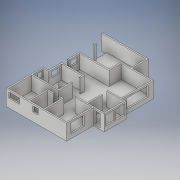
# Autodesk Inventor part: Erdgeschoss
Saved by Autodesk Inventor 2019 (Build 230136000, 136)
## iProperties
Created: 2019-04-30
Part Number: Erdgeschoss
Material: Generisch
Document SubType Name: Modeling
Designer: niede
Density: 1 g/cm^3
Appearance: Vorgabe
Author: niede
Autodesk Inventor part; units mm, degrees
ref_plane "YZ Plane" through (0, 0, 0) normal (1, 0, 0) x (0, 1, 0)
ref_plane "XZ Plane" through (0, 0, 0) normal (0, 1, 0) x (-1, 0, 0)
ref_plane "XY Plane" through (0, 0, 0) normal (0, 0, 1) x (1, 0, 0)
sketch "Skizze1" plane through (0, 0, 0) normal (0, 1, 0) x (-1, 0, 0)
  line L0 (0, 0) -> (11230, 0)
  line L1 (11230, 0) -> (11230, -6920)
  line L2 (11230, -6920) -> (10230, -6920)
  line L3 (10230, -6920) -> (10230, -17740)
  line L4 (10230, -17740) -> (11230, -17740)
  line L5 (11230, -17740) -> (11230, -17980)
  line L6 (11230, -17980) -> (2740, -17980)
  line L7 (2740, -17980) -> (2740, -14980)
  line L8 (2740, -14980) -> (-1250, -14980)
  line L9 (-1250, -14980) -> (-1250, -9110)
  line L10 (-1250, -9110) -> (-2000, -9110)
  line L11 (-2000, -9110) -> (-2000, -5010)
  line L12 (-2000, -5010) -> (0, -5010)
  line L13 (0, -5010) -> (0, 0)
  dimension "d0" = 11230
  dimension "d1" = 6920
  dimension "d2" = 1000
  dimension "d3" = 10820
  dimension "d4" = 1000
  dimension "d5" = 240
  dimension "d6" = 8490
  dimension "d11" = 3000
  dimension "d12" = 3990
  dimension "d13" = 5870
  dimension "d14" = 750
  dimension "d15" = 4100
  dimension "d16" = 2000
  constraints: 28 end point, 8 perpendicular, 2 point on line, 2 vertical, 1 horizontal
  measures "d0" distance of L0.start L0.end
  measures "d1" distance of L0.end L1.end
  measures "d2" distance of L1.end L2.end
  measures "d3" distance of L2.end L3.end
  measures "d4" distance of L3.end L4.end
  measures "d5" distance of L4.end L5.end
  measures "d6" distance of L5.end L6.end
  measures "d11" distance of L6.end L7.end
  measures "d12" distance of L7.end L8.end
  measures "d13" distance of L8.end L9.end
  measures "d14" distance of L9.end L10.end
  measures "d15" distance of L10.end L11.end
  measures "d16" distance of L11.end L12.end
extrude "Fundament" add sketch "Skizze1" along normal blind 300
sketch "Skizze3" plane through (0, 300, 0) normal (0, 1, 0) x (1, 0, 0)
  line L0 (0, 5010) -> (2000, 5010) projected
  line L1 (2000, 5010) -> (2000, 9110) projected
  line L2 (2000, 9110) -> (1250, 9110) projected
  line L3 (1250, 9110) -> (1250, 14980) projected
  line L4 (1250, 14980) -> (-2740, 14980) projected
  line L5 (-11230, 0) -> (0, 0)
  line L6 (0, 0) -> (0, 5010)
  line L7 (-240, 5010) -> (-1180.225, 5010)
  line L8 (-1180.225, 5250) -> (-1180.225, 7900)
  line L9 (-1180.225, 8900) -> (1250, 8900)
  line L10 (1250, 9110) -> (1250, 14980)
  line L11 (-2740, 14980) -> (-2740, 17980)
  line L12 (-2740, 17980) -> (-11230, 17980)
  line L13 (-10230, 6920) -> (-11230, 6920)
  line L14 (-11230, 6920) -> (-11230, 0)
  line L15 (-11230, 0) -> (-11230, 6920)
  line L16 (-11230, 0) -> (-11230, 6920)
  line L17 (-11230, 6920) -> (-10230, 6920)
  line L18 (-10230, 17740) -> (-11230, 17740)
  line L19 (-10230, 17740) -> (-11230, 17740)
  line L20 (-11230, 17980) -> (-2740, 17980)
  line L21 (-11230, 17740) -> (-11230, 17980)
  line L22 (-11230, 17980) -> (-2740, 17980)
  line L23 (-2740, 17980) -> (-2740, 14980)
  line L24 (1250, 14980) -> (1250, 9110)
  line L25 (-1180.225, 7900) -> (-1180.225, 5250)
  line L26 (0, 5010) -> (0, 0)
  line L27 (0, 0) -> (-11230, 0)
  line L28 (-240, 240) -> (-240, 5010)
  line L29 (-1420.225, 5250) -> (-1420.225, 7900)
  line L30 (-1420.225, 7900) -> (-1180.225, 7900)
  line L31 (-9990, 17740) -> (-6230, 17740)
  line L32 (-5990, 17740) -> (-2980, 17740)
  line L33 (-2980, 17740) -> (-2980, 14980)
  line L34 (-2980, 14740) -> (1010, 14740)
  line L35 (1010, 14740) -> (1010, 9140)
  line L36 (1010, 9140) -> (-1420.225, 9140)
  line L37 (-1420.225, 9140) -> (-1420.225, 8900)
  line L38 (-1420.225, 8900) -> (-952.7911, 8900)
  line L39 (-3420.225, 4770) -> (-3420.225, 5010)
  line L40 (-3420.225, 5010) -> (-2980, 5010)
  line L41 (-10990, 4530) -> (-6230, 4530)
  line L42 (-6230, 4530) -> (-5990, 4530)
  line L43 (-10990, 4770) -> (-6230, 4770)
  line L44 (-6990, 240) -> (-6990, 3530)
  line L45 (-6990, 3530) -> (-5990, 3530)
  line L46 (-5990, 3530) -> (-5990, 3770)
  line L47 (-5990, 3770) -> (-7230, 3770)
  line L48 (-7230, 3770) -> (-7230, 240)
  line L49 (-4480, 240) -> (-4480, 3530)
  line L50 (-4480, 3530) -> (-4990, 3530)
  line L51 (-4990, 3530) -> (-4990, 3770)
  line L52 (-4990, 3770) -> (-4240, 3770)
  line L53 (-4240, 3770) -> (-4240, 240)
  line L54 (-10990, 6680) -> (-9990, 6680)
  line L55 (-10230, 6920) -> (-10230, 17740) projected
  line L56 (-10230, 6920) -> (-10230, 9350)
  line L57 (-10230, 9350) -> (-5990, 9350)
  line L58 (-5990, 9350) -> (-5990, 8600)
  line L59 (-5990, 8600) -> (-6230, 8600)
  line L60 (-6230, 8600) -> (-6230, 9110)
  line L61 (-6230, 9110) -> (-9990, 9110)
  line L62 (-9990, 9110) -> (-9990, 6680)
  line L63 (-5990, 4530) -> (-5990, 7100)
  line L64 (-5990, 7100) -> (-5991.4024, 7100)
  line L65 (-5991.4024, 7100) -> (-5991.4024, 4770)
  line L66 (-8610, 4770) -> (-8610, 6270)
  line L67 (-8610, 6270) -> (-8370, 6270)
  line L68 (-8370, 6270) -> (-8370, 4770)
  line L69 (-6230, 6175) -> (-7370, 6175)
  line L70 (-7370, 6175) -> (-7370, 5935)
  line L71 (-7370, 5935) -> (-6230, 5935)
  line L72 (2000, 9110) -> (2000, 5010) projected
  line L73 (0, 5010) -> (2000, 5010)
  line L74 (2000, 5010) -> (2000, 9110)
  line L75 (1250, 9110) -> (2000, 9110) projected
  line L76 (2000, 9110) -> (1250, 9110)
  line L77 (-1180.225, 5010) -> (-1420.225, 5010)
  line L78 (-3420.225, 5010) -> (-3420.225, 5250)
  line L79 (-3420.225, 5250) -> (-1420.225, 5250)
  line L80 (-1420.225, 5010) -> (-3420.225, 5010)
  line L81 (1250, 8900) -> (1760, 8900)
  line L82 (1760, 8900) -> (1760, 5250)
  line L83 (1760, 5250) -> (-1180.225, 5250)
  line L84 (-2740, 14980) -> (1250, 14980)
  line L85 (-10230, 17740) -> (-10230, 6920) projected
  line L86 (-9990, 12449.8635) -> (-4540, 12449.8635)
  line L87 (-4540, 12449.8635) -> (-4540, 14740)
  line L88 (-4540, 14740) -> (-2980, 14740)
  line L89 (-10230, 12689.8635) -> (-4780, 12689.8635)
  line L90 (-4780, 12689.8635) -> (-4780, 14980)
  line L91 (-4780, 14980) -> (-2980, 14980)
  line L92 (-10230, 15189.8635) -> (-9990, 15189.8635)
  line L93 (-9990, 15189.8635) -> (-9990, 15589.8635)
  line L94 (-9990, 15589.8635) -> (-10230, 15589.8635)
  line L95 (-10230, 15589.8635) -> (-10230, 15189.8635)
  line L96 (-10230, 12449.8635) -> (-10230, 10350)
  line L97 (-9990, 10350) -> (-9990, 12449.8635)
  line L98 (-9990, 10350) -> (-10230, 10350)
  line L99 (-10990, 240) -> (-7230, 240)
  line L100 (-6990, 240) -> (-4480, 240)
  line L101 (-4240, 240) -> (-240, 240)
  line L102 (-10990, 240) -> (-10990, 4530)
  line L103 (-10990, 4770) -> (-10990, 6680)
  line L104 (-6230, 4770) -> (-6230, 5935)
  line L105 (-6230, 6175) -> (-6230, 7100)
  line L106 (-6230, 7100) -> (-5991.4024, 7100)
  line L107 (-10230, 12449.8635) -> (-10230, 12689.8635)
  line L108 (-9990, 17740) -> (-10230, 17740)
  line L109 (-5990, 17740) -> (-6230, 17740)
  dimension "d22" = 240
  dimension "d24" = 240
  dimension "d25" = 1000
  dimension "d26" = 240
  dimension "d27" = 240
  dimension "d28" = 240
  dimension "d30" = 240
  dimension "d31" = 240
  dimension "d33" = 240
  dimension "d42" = 240
  dimension "d43" = 240
  dimension "d44" = 240
  dimension "d45" = 240
  dimension "d47" = 2510
  dimension "d48" = 1000
  dimension "d49" = 1000
  dimension "d50" = 240
  dimension "d51" = 240
  dimension "d52" = 90
  dimension "d55" = 2202.7911
  dimension "d56" = 7480
  dimension "d57" = 2430
  dimension "d58" = 750
  dimension "d59" = 240
  dimension "d60" = 240
  dimension "d61" = 240
  dimension "d62" = 1500
  dimension "d63" = 1500
  dimension "d64" = 240
  dimension "d65" = 1000
  dimension "d66" = 240
  dimension "d67" = 240
  dimension "d68" = 240
  dimension "d69" = 240
  dimension "d70" = 240
  dimension "d71" = 5870
  dimension "d72" = 240
  dimension "d73" = 240
  dimension "d74" = 5690
  dimension "d75" = 240
  dimension "d76" = 5050.1365
  dimension "d77" = 2500
  dimension "d78" = 400
  dimension "d79" = 240
  dimension "d80" = 1000
  dimension "d81" = 90
  dimension "d82" = 90
  dimension "d83" = 90
  dimension "d84" = 30
  dimension "d85" = 3860
  dimension "d86" = 8870
  dimension "d87" = 9110
  dimension "d88" = 2010
  dimension "d89" = 5580
  dimension "d90" = 2935
  dimension "d91" = 2190
  dimension "d92" = 750
  dimension "d93" = 2000
  dimension "d94" = 3180.225
  dimension "d95" = 3420.225
  dimension "d96" = 4740
  dimension "d97" = 5420.225
  dimension "d98" = 6240
  dimension "d99" = 6540
  constraints: 202 end point, 50 perpendicular, 16 point on line, 9 horizontal, 8 collinear, 8 vertical, 6 parallel, 1 midpoint, 5 other
  measures "d22" distance between parallel lines of L6 L28
  measures "d24" distance between parallel lines of L8 L29
  measures "d25" distance between parallel lines of L30 L38
  measures "d26" distance between parallel lines of L9 L36
  measures "d27" distance of L9.start L37.end
  measures "d28" distance between parallel lines of L10 L35
  measures "d30" distance between parallel lines of L11 L33
  measures "d31" distance between parallel lines of L12 L32
  measures "d33" distance between parallel lines of L12 L31
  measures "d42" distance of L39.start L39.end
  measures "d43" distance between parallel lines of L53 L49
  measures "d44" distance between parallel lines of L44 L48
  measures "d45" distance between parallel lines of L47 L45
  measures "d47" distance between parallel lines of L44 L49
  measures "d48" distance of L50.end L45.end
  measures "d49" distance of L44.end L45.end
  measures "d50" distance between parallel lines of L43 L41
  measures "d51" distance between parallel lines of L13 L54
  measures "d52" angle of L40 L10
  measures "d55" distance from line of L38.end L10
  measures "d56" distance from line of L41.end L10
  measures "d57" distance of L55.start L56.end
  measures "d58" distance of L57.end L58.end
  measures "d59" distance between parallel lines of L57 L61
  measures "d60" distance between parallel lines of L56 L62
  measures "d61" distance between parallel lines of L60 L58
  measures "d62" distance of L58.end L63.end
  measures "d63" distance of L66.start L66.end
  measures "d64" distance of L66.end L67.end
  measures "d65" distance between parallel lines of L68 L70
  measures "d66" distance between parallel lines of L69 L71
  measures "d67" distance of L39.end L78.end
  measures "d68" distance between parallel lines of L0 L83
  measures "d69" distance between parallel lines of L1 L82
  measures "d70" distance between parallel lines of L4 L34
  measures "d71" distance of L24.start L10.start
  measures "d72" distance between parallel lines of L91 L88
  measures "d73" distance between parallel lines of L87 L90
  measures "d74" distance of L96.start L86.end
  measures "d75" distance between parallel lines of L86 L89
  measures "d76" distance between parallel lines of L31 L89
  measures "d77" distance between parallel lines of L89 L92
  measures "d78" distance of L92.end L93.end
  measures "d79" distance of L92.start L92.end
  measures "d80" distance between parallel lines of L57 L98
  measures "d81" angle of L1 L7
  measures "d82" angle of L75 L39
  measures "d83" angle of L75 L21
  measures "d84" distance between parallel lines of L2 L36
  measures "d85" distance between parallel lines of L2 L79
  measures "d86" distance between parallel lines of L2 L12
  measures "d87" distance between parallel lines of L2 L27
  measures "d88" distance between parallel lines of L2 L64
  measures "d89" distance between parallel lines of L2 L45
  measures "d90" distance between parallel lines of L2 L69
  measures "d91" distance between parallel lines of L2 L13
  measures "d92" distance between parallel lines of L72 L10
  measures "d93" distance between parallel lines of L72 L26
  measures "d94" distance between parallel lines of L72 L8
  measures "d95" distance between parallel lines of L72 L37
  measures "d96" distance between parallel lines of L72 L23
  measures "d97" distance between parallel lines of L72 L78
  measures "d98" distance between parallel lines of L72 L53
  measures "d99" distance between parallel lines of L72 L87
extrude "Wände" add sketch "Skizze3" along normal blind 2600 contours L6 L5 L14 L13 L55 L57 L58 L59 L60 L61 L62 L54 L103 L43 L104 L71 L70 L69 L105 L106 L64 L63 L42 L41 L102 L99 L48 L47 L46 L45 L44 L100 L49 L50 L51 L52 L53 L101 L28 L7 L77 L80 L40 L78 L79 L29 L30 L8 L83 L82 L81 L9 L38 L37 L36 L35 L34 L88 L87 L86 L97 L98 L89 L90 L91 L33 L32 L109 L31 L108 L18 L21 L12 L11 L4 L3 L2 L1 L0 | L55 L94 L93 L92
sketch "Skizze4" plane through (-11230, 0, 0) normal (0, 0, 1) x (1, 0, 0)
  line L0 (500, 2600) -> (2500, 2600)
  line L1 (2500, 2600) -> (2500, 1600)
  line L2 (2500, 1600) -> (500, 1600)
  line L3 (500, 1600) -> (500, 2600)
  line L4 (5000, 2600) -> (6000, 2600)
  line L5 (6000, 2600) -> (6000, 1600)
  line L6 (6000, 1600) -> (5000, 1600)
  line L7 (5000, 1600) -> (5000, 2600)
  line L8 (0, 2900) -> (11230, 2900) projected
  line L9 (0, 0) -> (0, 2900) projected
  dimension "d191" = 2500
  dimension "d192" = 1000
  dimension "d193" = 300
  dimension "d194" = 1000
  dimension "d195" = 2000
  dimension "d196" = 500
  constraints: 16 end point, 4 parallel, 2 horizontal, 2 perpendicular, 2 point on line
  measures "d191" distance between parallel lines of L7 L1
  measures "d192" distance of L2.end L0.start
  measures "d193" distance between parallel lines of L8 L4
  measures "d194" distance of L5.end L6.end
  measures "d195" distance of L1.end L2.end
  measures "d196" distance between parallel lines of L9 L3
extrude "Fenster_West" cut sketch "Skizze4" against normal blind 240
sketch "Skizze5" plane through (0, 0, 0) normal (1, 0, 0) x (0, 0, -1)
  line L0 (0, 2900) -> (5010, 2900) projected
  line L1 (0, 0) -> (0, 2900) projected
  line L2 (800, 2600) -> (3300, 2600)
  line L3 (3300, 2600) -> (3300, 800)
  line L4 (3300, 800) -> (800, 800)
  line L5 (800, 800) -> (800, 2600)
  dimension "d140" = 800
  dimension "d141" = 300
  dimension "d142" = 1800
  dimension "d143" = 2500
  constraints: 8 end point, 2 parallel, 1 horizontal, 1 perpendicular
  measures "d140" distance between parallel lines of L1 L5
  measures "d141" distance between parallel lines of L0 L2
  measures "d142" distance of L4.end L2.start
  measures "d143" distance of L3.end L4.end
extrude "Fenster_Süd_1" cut sketch "Skizze5" against normal blind 240
sketch "Skizze6" plane through (1250, 0, -9110) normal (1, 0, 0) x (0, 0, -1)
  line L0 (830, 2600) -> (4830, 2600)
  line L1 (4830, 2600) -> (4830, 800)
  line L2 (4830, 800) -> (830, 800)
  line L3 (830, 800) -> (830, 2600)
  line L4 (30, 300) -> (30, 2900) projected
  line L5 (0, 2900) -> (5870, 2900) projected
  point P0 (-9110, 0)
  dimension "d146" = 800
  dimension "d147" = 1800
  dimension "d148" = 4000
  dimension "d197" = 300
  constraints: 8 end point, 2 parallel, 1 horizontal, 1 perpendicular
  measures "d146" distance between parallel lines of L4 L3
  measures "d147" distance of L2.end L0.start
  measures "d148" distance of L1.end L2.end
  measures "d197" distance between parallel lines of L5 L0
extrude "Fenster_Süd_2" cut sketch "Skizze6" against normal blind 240
sketch "Skizze7" plane through (0, 0, -5010) normal (0, 0, 1) x (1, 0, 0)
  line L0 (0, 2900) -> (2000, 2900) projected
  line L1 (0, 0) -> (0, 2900) projected
  line L2 (250, 2600) -> (1250, 2600)
  line L3 (1250, 2600) -> (1250, 300)
  line L4 (1250, 300) -> (250, 300)
  line L5 (250, 300) -> (250, 2600)
  line L6 (-1180.225, 300) -> (1760, 300) projected
  dimension "d162" = 250
  dimension "d163" = 1000
  dimension "d165" = 300
  constraints: 8 end point, 2 parallel, 1 collinear, 1 horizontal, 1 perpendicular
  measures "d162" distance between parallel lines of L1 L5
  measures "d163" distance of L2.start L2.end
  measures "d165" distance between parallel lines of L0 L2
extrude "Fenster_Wintergarten_1" cut sketch "Skizze7" against normal blind 240
sketch "Skizze8" plane through (2000, 0, -5010) normal (1, 0, 0) x (0, 0, -1)
  line L0 (4100, 0) -> (4100, 2900) projected
  line L1 (0, 2900) -> (4100, 2900) projected
  line L2 (0, 0) -> (0, 2900) projected
  line L3 (240, 2600) -> (1930, 2600)
  line L4 (1930, 2600) -> (1930, 800)
  line L5 (1930, 800) -> (240, 800)
  line L6 (240, 800) -> (240, 2600)
  line L7 (2170, 2600) -> (3860, 2600)
  line L8 (3860, 2600) -> (3860, 800)
  line L9 (3860, 800) -> (2170, 800)
  line L10 (2170, 800) -> (2170, 2600)
  point P0 (-5010, 0)
  dimension "d168" = 240
  dimension "d169" = 240
  dimension "d170" = 240
  dimension "d171" = 1690
  dimension "d172" = 1800
  dimension "d173" = 1800
  dimension "d174" = 300
  constraints: 16 end point, 4 parallel, 2 horizontal, 2 perpendicular, 1 point on line
  measures "d168" distance between parallel lines of L10 L4
  measures "d169" distance between parallel lines of L2 L6
  measures "d170" distance between parallel lines of L0 L8
  measures "d171" distance of L7.start L7.end
  measures "d172" distance of L5.end L3.start
  measures "d173" distance of L7.end L8.end
  measures "d174" distance between parallel lines of L1 L3
extrude "Fenster_Wintergarten_2" cut sketch "Skizze8" against normal blind 240
sketch "Skizze9" plane through (-10230, 0, -17740) normal (-1, 0, 0) x (0, 0, 1)
  line L0 (10820, 0) -> (10820, 2900) projected
  line L1 (7390, 300) -> (7390, 2900) projected
  line L2 (5050.1365, 2900) -> (7390, 2900) projected
  line L3 (5690, 2600) -> (7090, 2600)
  line L4 (7090, 2600) -> (7090, 1600)
  line L5 (7090, 1600) -> (5690, 1600)
  line L6 (5690, 1600) -> (5690, 2600)
  line L7 (9120, 2600) -> (10520, 2600)
  line L8 (10520, 2600) -> (10520, 1600)
  line L9 (10520, 1600) -> (9120, 1600)
  line L10 (9120, 1600) -> (9120, 2600)
  point P0 (17740, 0)
  dimension "d177" = 300
  dimension "d178" = 1000
  dimension "d179" = 300
  dimension "d180" = 1400
  dimension "d181" = 300
  dimension "d182" = 1400
  constraints: 16 end point, 4 parallel, 2 horizontal, 2 perpendicular, 2 point on line
  measures "d177" distance between parallel lines of L1 L4
  measures "d178" distance of L9.end L7.start
  measures "d179" distance between parallel lines of L2 L3
  measures "d180" distance of L8.end L9.end
  measures "d181" distance between parallel lines of L0 L8
  measures "d182" distance of L4.end L5.end
extrude "Fenster_Nord" cut sketch "Skizze9" against normal blind 240
sketch "Skizze10" plane through (-11230, 0, -6920) normal (-1, 0, 0) x (0, 0, 1)
  line L0 (0, 2900) -> (6920, 2900) projected
  line L1 (0, 0) -> (0, 2900) projected
  line L2 (300, 2600) -> (1300, 2600)
  line L3 (1300, 2600) -> (1300, 1600)
  line L4 (1300, 1600) -> (300, 1600)
  line L5 (300, 1600) -> (300, 2600)
  dimension "d185" = 300
  dimension "d186" = 300
  dimension "d187" = 1000
  dimension "d188" = 1000
  constraints: 8 end point, 2 parallel, 1 horizontal, 1 perpendicular
  measures "d185" distance between parallel lines of L1 L5
  measures "d186" distance between parallel lines of L0 L2
  measures "d187" distance of L2.end L3.end
  measures "d188" distance of L3.end L4.end
extrude "Fenster_Wäscheraum" cut sketch "Skizze10" against normal blind 240
